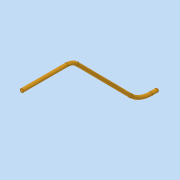
# Autodesk Inventor part: 2mmToRudder
Saved by Autodesk Inventor 2017 (Build 210142000, 142)
## iProperties
Created: 2016-12-11
Part Number: 2mmToRudder
Material: Brass, Soft Yellow, Welded
Document SubType Name: Modeling
Designer: techn
Density: 8.5 g/cm^3
Appearance: Weld - Brass
Author: techn
Autodesk Inventor part; units mm, degrees
ref_plane "YZ Plane" through (0, 0, 0) normal (1, 0, 0) x (0, 1, 0)
ref_plane "XZ Plane" through (0, 0, 0) normal (0, 1, 0) x (-1, 0, 0)
ref_plane "XY Plane" through (0, 0, 0) normal (0, 0, 1) x (1, 0, 0)
sketch "Sketch2" plane through (0, 0, 0) normal (1, 0, 0) x (0, 1, 0)
  line L0 (0, 0) -> (0, -25.4)
  arc A0 (-2.4205, -31.1983) -> (0, -25.4) centre (-8.1552, -25.4) ccw
  line L1 (-2.4205, -31.1983) -> (-33.2771, -61.7168)
  arc A1 (-33.2771, -61.7168) -> (-38.1, -73.2701) centre (-21.8504, -73.2701) ccw
  line L2 (-38.1, -73.2701) -> (-38.1, -76.4451)
  dimension "d3" = 25.4
  dimension "d4" = 8.1552
  dimension "d5" = 16.2496
  dimension "d6" = 3.175
  dimension "d7" = 38.1
  constraints: 6 end point, 4 point on circle, 4 tangent, 2 centre point, 2 vertical
  measures "d3" distance of L0.start L0.end
  measures "d4" radius of A0
  measures "d5" radius of A1
  measures "d6" distance of L2.start L2.end
  measures "d7" distance between parallel lines of L0 L2
sketch "Sketch3" plane through (0, 0, 0) normal (0, 0, 1) x (1, 0, 0)
  circle A0 centre (0, 0) radius 1
  dimension "d8" = 2
  constraints: 1 centre point, 1 coincident
  measures "d8" diameter of A0
sweep "Sweep1" add profiles "Sketch3" path "Sketch2"
sketch "Sketch4" plane through (0, 0, 0) normal (1, 0, 0) x (0, 1, 0)
  line L0 (-39.1, -76.4451) -> (-37.1, -76.4451) projected
  line L1 (-37.1, -73.2701) -> (-37.1, -76.4451) projected
  arc A0 (-39.1, -76.4451) -> (-37.1, -76.4451) centre (-38.1, -76.4451) ccw
  point P0 (0, 0)
  constraints: 2 point on circle, 1 centre point, 1 tangent
revolve "Revolution1" add sketch "Sketch4" angle 180 mid plane about axis through (0, -39.1, -76.4451) along (0, 1, 0)
body "Solid2"
